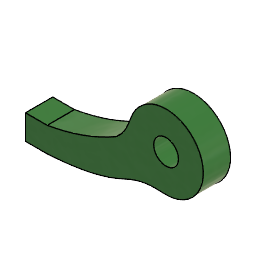
Lever assembly version 2 (Autodesk Fusion 360 archive; units mm, degrees)
design "Arm for lever (version 2)"
part number: 2026-04-11-21-13-19-627
Autodesk Fusion 360 part; units mm, degrees
sketch "Sketch1" plane through (0, 0, 0) normal (0, 1, 0) x (1, 0, 0)
  line L0 (25.4, 0) -> (25.4, -25.4)
  line L1 (0, 0) -> (0, -6.35)
  spline S0 degree 5 poles (0, -6.35) (0.5329, -6.444) (1.5966, -6.6439) (3.1854, -6.9795) (5.2905, -7.4995) (7.8979, -8.2785) (10.4794, -9.1975) (13.033, -10.2671) (15.5578, -11.4919) (18.0554, -12.8641) (20.5278, -14.3719) (22.4874, -15.6774) (23.9474, -16.7087) (24.9165, -17.4191) (25.4, -17.78) knots 0 0 0 0 0 0 0.1 0.2 0.3 0.4 0.5 0.6 0.7 0.8 0.9 1 1 1 1 1 1
  spline S1 degree 5 poles (0, 0) (0.6299, -0.0379) (1.8795, -0.1233) (3.723, -0.2806) (6.1181, -0.5492) (8.9998, -0.9904) (11.7581, -1.5473) (14.3813, -2.2312) (16.8599, -3.0508) (19.195, -4.0053) (21.3952, -5.0863) (23.0555, -6.045) (24.248, -6.8135) (25.0198, -7.3476) (25.4, -7.62) knots 0 0 0 0 0 0 0.1 0.2 0.3 0.4 0.5 0.6 0.7 0.8 0.9 1 1 1 1 1 1
  circle A0 centre (30.4647, -15.6868) radius 9.525
  spline S2 degree 5 poles (20.0465, -4.4483) (20.2591, -4.5455) (20.683, -4.7339) (21.315, -4.9982) (22.1502, -5.3135) (23.1806, -5.642) (24.1963, -5.9) (25.1959, -6.0844) (26.1788, -6.196) (27.1456, -6.2452) (28.0979, -6.2481) (28.8493, -6.2266) (29.4075, -6.2031) (29.7774, -6.1849) (29.9618, -6.1751) knots 0 0 0 0 0 0 0.1 0.2 0.3 0.4 0.5 0.6 0.7 0.8 0.9 1 1 1 1 1 1
  spline S3 degree 5 poles (17.7046, -12.7) (17.8079, -12.7855) (18.0118, -12.9599) (18.3094, -13.2317) (18.6897, -13.6147) (19.1358, -14.13) (19.5506, -14.6847) (19.9329, -15.2812) (20.2836, -15.9198) (20.6073, -16.5969) (20.9096, -17.3077) (21.139, -17.8995) (21.306, -18.3549) (21.4153, -18.6634) (21.4694, -18.8189) knots 0 0 0 0 0 0 0.1 0.2 0.3 0.4 0.5 0.6 0.7 0.8 0.9 1 1 1 1 1 1
  circle A1 centre (30.4647, -15.6868) radius 3.175
  point P0 (12.7, -10.16)
  point P1 (15.24, -2.54)
  point P2 (25.4, -6.096)
  point P3 (19.8566, -15.1781)
  dimension "d1" = 6.35
  dimension "d2" = 19.05
  dimension "d3" = 6.35
  constraint vertical L0
  constraint coincident L1.start S1.start
  constraint vertical L1
  constraint coincident L0 S0.end
  constraint coincident L0 S1.end
  constraint coincident S1.end A0
  constraint coincident S1 S2.start
  constraint coincident L0 P2
  constraint coincident A0 S2.end
  constraint coincident S0 S3.start
  constraint coincident A0 S3.end
  constraint tangent A0 S3
  constraint tangent A0 S2
  constraint concentric A0 A1
  measures "d1" distance of L1.start L1.end
  measures "d2" diameter of A0
  measures "d3" diameter of A1
extrude "Extrude1" add sketch "Sketch1" along normal blind 7.0104
extrude "Extrude2" add 1 faces at (0, 2.3368, 2.1167) along direction (-1, 0, 0) blind 5.588

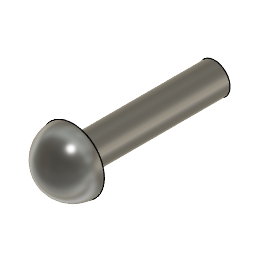
design "Axel"
part number: 2026-04-09-19-47-45-566
Autodesk Fusion 360 part; units mm, degrees
sketch "Sketch1" plane through (0, 0, 0) normal (0, 1, 0) x (1, 0, 0)
  circle A0 centre (0, 0) radius 3.1115
  dimension "d1" = 6.223
  constraint coincident A0.centre origin
  measures "d1" diameter of A0
extrude "Extrude1" add sketch "Sketch1" along normal blind 19.05
sketch "Sketch2" plane through (0, 0, 0) normal (0, -1, 0) x (1, 0, 0)
  circle A0 centre (0, 0) radius 3.1115
  circle A1 centre (0, 0) radius 6.35
  dimension "d4" = 12.7
  constraint concentric A0 A1
  measures "d4" diameter of A1
extrude "Extrude2" add sketch "Sketch2" along normal blind 6.35 contours A0 | A1
fillet "Fillet1" radius 6.35 1 edges at (-5.9203, -6.35, -2.2963)
extrude "Extrude3" add 1 faces at (-1.7613, 19.05, -0.2234) along direction (0, 1, 0) blind 25.4
extrude "Extrude4" cut 1 faces at (-1.7613, 44.45, -0.2234) along direction (0, -1, 0) blind 7.62
extrude "Extrude5" cut 1 faces at (-1.7613, 36.83, -0.2234) along direction (0, -1, 0) blind 8.255

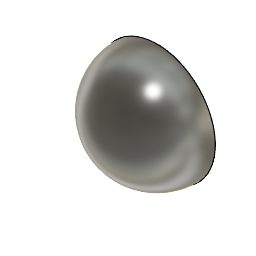
design "Peg topper"
part number: 2026-04-09-20-01-08-332
Autodesk Fusion 360 part; units mm, degrees
sketch "Sketch1" plane through (0, 0, 0) normal (0, 1, 0) x (1, 0, 0)
  circle A0 centre (0, 0) radius 6.35
  dimension "d1" = 12.7
  constraint coincident A0.centre origin
  measures "d1" diameter of A0
extrude "Extrude1" add sketch "Sketch1" along normal blind 6.35
fillet "Fillet1" radius 6.35 1 edges at (-5.9203, 0, 2.2963)
